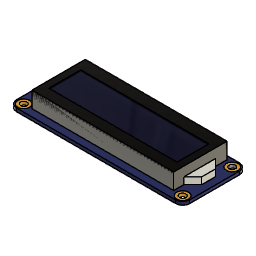
LCD1602 RGB Module v1 (Autodesk Fusion 360 design; units mm, degrees)
Autodesk Fusion 360 part; units mm, degrees
sketch "Skizze1" plane through (0, 0, 0) normal (0, 0, 1) x (1, 0, 0) in component "i2c display"
  circle A0 centre (0, 0) radius 3.6
  circle A1 centre (0, 25) radius 3.6
  circle A2 centre (80, 25) radius 3.6
  circle A3 centre (80, 0) radius 3.6
  line L0 (0, -3.6) -> (80, -3.6)
  line L1 (-3.6, 0) -> (-3.6, 25)
  line L2 (0, 28.6) -> (80, 28.6)
  line L3 (83.6, 25) -> (83.6, 0)
  line L4 (4.2, 0) -> (75.5, 0)
  line L5 (75.5, 0) -> (75.5, 26.8)
  line L6 (75.5, 26.8) -> (4.2, 26.8)
  line L7 (4.2, 26.8) -> (4.2, 0)
  line L8 (7.6, 21.1) -> (72.1, 21.1)
  line L9 (72.1, 21.1) -> (72.1, 5.1)
  line L10 (72.1, 5.1) -> (7.6, 5.1)
  line L11 (7.6, 5.1) -> (7.6, 21.1)
  circle A4 centre (0, 0) radius 3
  circle A5 centre (0, 25) radius 3
  circle A6 centre (80, 25) radius 3
  circle A7 centre (80, 0) radius 3
  circle A8 centre (0, 25) radius 1.6
  circle A9 centre (0, 0) radius 1.6
  circle A10 centre (80, 25) radius 1.6
  circle A11 centre (80, 0) radius 1.6
  line L12 (75.5, 5.1) -> (80, 9.6)
  line L13 (75.5, 5.1) -> (81.864, 5.1) construction
  line L14 (75.5, 21.1) -> (80, 16.6)
  line L15 (80, 16.6) -> (80, 9.6)
  dimension "d1" = 7.2
  dimension "d2" = 7.2
  dimension "d3" = 80
  dimension "d5" = 7.2
  dimension "d6" = 7.2
  dimension "d8" = 7.8
  dimension "d9" = 71.3
  dimension "d10" = 26.8
  dimension "d14" = 64.5
  dimension "d15" = 16
  dimension "d16" = 6
  dimension "d17" = 6
  dimension "d18" = 6
  dimension "d19" = 6
  dimension "d20" = 3.2
  dimension "d21" = 3.2
  dimension "d22" = 3.2
  dimension "d23" = 3.2
  dimension "d32" = 45
  dimension "d33" = 90
  constraint coincident A0.centre A4.centre
  constraint coincident A0 L0.start
  constraint coincident A3 L0.end
  constraint tangent A3 L0
  constraint horizontal L0
  constraint coincident A0 L1.start
  constraint coincident A1 L1.end
  constraint tangent A1 L1
  constraint coincident A1 L2.start
  constraint coincident A2 L2.end
  constraint tangent A2 L2
  constraint coincident A2 L3.start
  constraint coincident A3 L3.end
  constraint tangent A3 L3
  constraint parallel L1 L3
  constraint horizontal L4
  constraint vertical L5
  constraint horizontal L6
  constraint vertical L7
  constraint horizontal L8
  constraint vertical L9
  constraint horizontal L10
  constraint vertical L11
  constraint concentric A1 A5
  constraint concentric A2 A6
  constraint concentric A3 A7
  constraint concentric A5 A8
  constraint concentric A0 A9
  constraint concentric A2 A10
  constraint concentric A3 A11
  constraint coincident L5 L14.start
  constraint coincident L5 L12.start
  constraint horizontal L13
  constraint parallel L5 L15
  measures "d1" diameter of A0
  measures "d2" diameter of A1
  measures "d3" distance of A0.centre A3.centre
  measures "d5" diameter of A2
  measures "d6" diameter of A3
  measures "d8" distance of L1.start L4.start
  measures "d9" distance of L4.start L4.end
  measures "d10" distance of L4.start L6.end
  measures "d14" distance of L8.start L8.end
  measures "d15" distance of L8.start L10.end
  measures "d16" diameter of A4
  measures "d17" diameter of A5
  measures "d18" diameter of A6
  measures "d19" diameter of A7
  measures "d20" diameter of A8
  measures "d21" diameter of A9
  measures "d22" diameter of A10
  measures "d23" diameter of A11
  measures "d32" angle of L12 L13
  measures "d33" angle of L12 L14
extrude "Extrusion1" add sketch "Skizze1" along normal blind 1.6 contours A0 | A0 A1 A2 A3 L0 L1 L2 L3 | A1 | A3 | A2 | L5 L12 L14 L15 makes body 1 in component "i2c display"
extrude "Extrusion2" add sketch "Skizze1" along normal blind 1.6 separate body contours A4 | A5 | A6 | A7 makes body 2 at (2.9851, -0.2987, 1.0667) makes body 3 at (78.6314, -2.6696, 0.5333) makes body 4 at (2.9851, 24.7013, 1.0667) makes body 5 at (82.9851, 24.7013, 1.0667) in component "i2c display"
extrude "Extrusion3" add sketch "Skizze1" along normal blind 9.7 contours L4 L5 L6 L7 bodies 1 in component "i2c display"
extrude "Extrusion4" add sketch "Skizze1" along normal blind 9.5 contours L8 L9 L10 L11 bodies 1 in component "i2c display"
extrude "Extrusion5" add sketch "Skizze1" along normal blind 3.5 separate body contours L5 L12 L14 L15 makes body 6 in component "i2c display"
extrude "Extrusion6" add 1 faces at (77, 14.2667, 3.5) along direction (0, 0, 1) blind 0.5 on bodies 6 bodies 6 2 3 4 5 1 in component "i2c display"
extrude "Extrusion7" add 1 faces at (77, 14.2667, 4) along direction (0, 0, 1) blind 1 on bodies 6 bodies 6 in component "i2c display"
extrude "Extrusion8" add sketch "Skizze1" along normal blind 9 separate body contours L8 L9 L10 L11 makes body 7 in component "i2c display"
extrude "Extrusion9" add sketch "Skizze1" along normal blind 9.7 separate body contours L4 L5 L6 L7 makes body 8 in component "i2c display"
component "i2c display" placed x (1, 0, 0) y (0, 1, 0) z (0, 0, 1) at (0, 0, 0)
